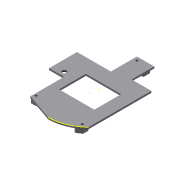
# Autodesk Inventor part: Raman2Go_Adapterplatte1_XY-TischChina
Saved by Autodesk Inventor 2019 (Build 230136000, 136)
## iProperties
Created: 2018-09-10
Part Number: Raman2Go_Adapterplatte1_XY-TischChina
Material: Generisch
Document SubType Name: Modeling
Designer: Henry John
Density: 1 g/cm^3
Appearance: Vorgabe
Author: Henry John
Autodesk Inventor part; units mm, degrees
ref_plane "YZ Plane" through (0, 0, 0) normal (1, 0, 0) x (0, 1, 0)
ref_plane "XZ Plane" through (0, 0, 0) normal (0, 1, 0) x (-1, 0, 0)
ref_plane "XY Plane" through (0, 0, 0) normal (0, 0, 1) x (1, 0, 0)
sketch "Skizze1" plane through (0, 0, 0) normal (0, 0, 1) x (1, 0, 0)
  circle A0 centre (-18.8292, -0.8203) radius 1.45 construction
  line L0 (-24.8792, -2.7703) -> (-24.8792, 8.6797) construction
  arc A1 (-11.8792, -25.2203) -> (6.3208, -26.6782) centre (-1.0025, -3.77) ccw construction
  circle A2 centre (-14.9792, -20.5703) radius 0.9 construction
  circle A3 centre (12.0208, -21.4394) radius 0.9 construction
  circle A4 centre (-3.6792, 25.2797) radius 0.9 construction
  line L1 (-5.6792, 27.2797) -> (3.4208, 27.2797) construction
  line L2 (25.1208, 7.4797) -> (25.1208, -1.5203) construction
  line L3 (25.1208, -27.8203) -> (-24.8792, -27.8203)
  line L4 (-24.8792, -27.8203) -> (-24.8792, 27.2797)
  line L5 (-24.8792, 27.2797) -> (25.1208, 27.2797)
  line L6 (25.1208, 27.2797) -> (25.1208, -27.8203)
  line L7 (4.6208, 0.2797) -> (4.6208, -6.9703) construction
  line L8 (-4.8792, 0.2797) -> (4.6208, 0.2797) construction
  line L9 (-4.8792, -6.9703) -> (-4.8792, 0.2797) construction
  line L10 (4.6208, -6.9703) -> (-4.8792, -6.9703) construction
  line L11 (-2.2292, 2.2797) -> (1.9708, 2.2797) construction
  line L12 (6.3708, 2.2797) -> (1.9708, 2.2797) construction
  line L13 (6.3708, -8.9703) -> (6.3708, 2.2797) construction
  line L14 (1.9708, -8.9703) -> (6.3708, -8.9703) construction
  line L15 (1.9708, -8.9703) -> (-2.2292, -8.9703) construction
  line L16 (-6.6292, -8.9703) -> (-2.2292, -8.9703) construction
  line L17 (-6.6292, 2.2797) -> (-6.6292, -8.9703) construction
  line L18 (-2.2292, 2.2797) -> (-6.6292, 2.2797) construction
  line L19 (-11.6292, -10.9703) -> (8.3708, -10.9703)
  line L20 (8.3708, -10.9703) -> (8.3708, 4.2797)
  line L21 (8.3708, 4.2797) -> (-11.6292, 4.2797)
  line L22 (-11.6292, 4.2797) -> (-11.6292, -10.9703)
  point P0 (0, 0)
  dimension "d48" = 2
  dimension "d49" = 2
  dimension "d50" = 2
  dimension "d51" = 5
  constraints: 16 end point, 4 parallel, 3 collinear, 2 horizontal, 2 perpendicular, 1 tangent
  measures "d48" distance between parallel lines of L20 L13
  measures "d49" distance between parallel lines of L18 L21
  measures "d50" distance between parallel lines of L15 L19
  measures "d51" distance between parallel lines of L17 L22
extrude "Extrusion1" add sketch "Skizze1" along normal blind 1
sketch "Skizze2" plane through (0, 0, 0) normal (0, 0, -1) x (-1, 0, 0)
  circle A0 centre (14.9792, -20.5703) radius 0.9 projected
  circle A1 centre (-12.0208, -21.4394) radius 0.9 construction
  circle A2 centre (3.6792, 25.2797) radius 0.9 construction
  circle A3 centre (14.9792, -20.5703) radius 0.9 projected
  circle A4 centre (9.7292, -19.9703) radius 0.75 projected
  line L0 (17.9792, -20.8203) -> (16.3292, -20.8203) construction
  line L1 (7.7292, -22.4703) -> (11.8792, -22.4703) construction
  line L2 (7.7292, -17.4703) -> (7.7292, -22.4703) construction
  line L3 (16.3292, -17.4703) -> (7.7292, -17.4703) construction
  line L4 (16.3292, -20.8203) -> (16.3292, -17.4703) construction
  line L5 (16.3292, -22.2703) -> (7.9292, -22.2703)
  line L6 (7.9292, -22.2703) -> (7.9292, -17.6703)
  line L7 (7.9292, -17.6703) -> (16.3292, -17.6703)
  line L8 (16.3292, -17.6703) -> (16.3292, -22.2703)
  line L9 (11.8792, -22.2703) -> (12.162, -22.2703) construction
  line L10 (16.3292, -17.6703) -> (12.3496, -17.6703)
  line L11 (12.3496, -17.6703) -> (12.3496, -22.2703)
  line L12 (12.3496, -22.2703) -> (16.3292, -22.2703)
  line L13 (16.3292, -22.2703) -> (16.3292, -17.6703)
  line L14 (16.3292, -22.2703) -> (13.494, -22.2703)
  line L15 (13.494, -22.2703) -> (13.494, -18.9379)
  line L16 (13.494, -18.9379) -> (16.3292, -18.9379)
  line L17 (16.3292, -18.9379) -> (16.3292, -22.2703)
  point P0 (0, 0)
  dimension "d3" = 0.2
  dimension "d4" = 0.2
  dimension "d9" = 0.2
  constraints: 26 end point, 5 parallel, 4 point on line, 3 horizontal, 2 perpendicular, 2 vertical, 1 vertical alignment
  measures "d3" distance between parallel lines of L3 L7
  measures "d4" distance between parallel lines of L2 L6
  measures "d9" distance between parallel lines of L5 L1
extrude "Extrusion2" add sketch "Skizze2" along normal blind 2.5 contours A0 | L5 L15 L16 L8
sketch "Skizze3" plane through (0, 0, -2.5) normal (0, 0, -1) x (-1, 0, 0)
  circle A0 centre (14.9792, -20.5703) radius 0.9 construction
  point P0 (0, 0)
hole "Bohrung1" at (-14.9792, -20.5703, -2.5) direction (0, 0, 1) diameter 1.221 depth 6.1 tip angle 118 thread size "M1.6x0.35" class "6H" standard "ISO Metric profile"
sketch "Skizze4" plane through (0, 0, 0) normal (0, 0, -1) x (-1, 0, 0)
  circle A0 centre (18.8292, -0.8203) radius 1.45 construction
  point P0 (0, 0)
hole "Bohrung2" at (-18.8292, -0.8203, 0) direction (0, 0, 1) diameter 2.459 end through all thread size "M3x0.5" class "6H" standard "ISO Metric profile"
sketch "Skizze5" plane through (0, 0, 0) normal (0, 0, -1) x (-1, 0, 0)
  line L0 (-9.3708, -21.4703) -> (-9.3708, -17.9703) construction
  line L1 (-14.1208, -16.9703) -> (-14.1208, -22.4703) construction
  line L2 (-15.3208, -16.9703) -> (-10.3708, -16.9703) construction
  line L3 (-9.3708, -17.9703) -> (-10.3708, -16.9703) construction
  line L4 (-9.3708, -21.4703) -> (-9.3708, -17.9703) construction
  line L5 (-10.5708, -16.9703) -> (-15.3208, -16.9703)
  line L6 (-15.3208, -16.9703) -> (-15.3208, -24.3394)
  line L7 (-15.3208, -24.3394) -> (-10.5708, -24.3394)
  line L8 (-10.5708, -24.3394) -> (-10.5708, -16.9703)
  line L9 (-15.3208, -16.9703) -> (-15.3208, -1.5203) construction
  circle A0 centre (-12.0208, -21.4394) radius 0.9 construction
  line L10 (-10.5708, -24.3394) -> (-13.7279, -24.3394)
  line L11 (-13.7279, -24.3394) -> (-13.7279, -16.9703)
  line L12 (-13.7279, -16.9703) -> (-10.5708, -16.9703)
  line L13 (-10.5708, -16.9703) -> (-10.5708, -24.3394)
  line L14 (-10.5708, -24.3394) -> (-13.7279, -24.3394)
  line L15 (-13.7279, -24.3394) -> (-13.7279, -19.7203)
  line L16 (-13.7279, -19.7203) -> (-10.5708, -19.7203)
  line L17 (-10.5708, -19.7203) -> (-10.5708, -24.3394)
  point P0 (0, 0)
extrude "Extrusion3" add sketch "Skizze5" along normal blind 2.3 contours L8 L7 L11 L16
sketch "Skizze6" plane through (0, 0, -2.3) normal (0, 0, -1) x (-1, 0, 0)
  circle A0 centre (-12.0208, -21.4394) radius 0.9 construction
  point P0 (0, 0)
hole "Bohrung3" at (12.0208, -21.4394, -2.3) direction (0, 0, 1) diameter 1.221 depth 7.1 tip angle 118 thread size "M1.6x0.35" class "6H" standard "ISO Metric profile"
sketch "Skizze7" plane through (0, 0, 0) normal (0, 0, -1) x (-1, 0, 0)
  circle A0 centre (3.6792, 25.2797) radius 0.9 construction
  line L0 (-3.4208, 24.7797) -> (-3.4208, 27.2797) construction
  line L1 (-1.9208, 24.7797) -> (-3.4208, 24.7797) construction
  line L2 (-1.9208, 23.2797) -> (-1.9208, 24.7797) construction
  line L3 (5.6792, 23.2797) -> (-1.9208, 23.2797) construction
  line L4 (5.6792, 27.2797) -> (5.6792, 23.2797) construction
  line L5 (-3.4208, 27.2797) -> (5.6792, 27.2797) construction
  line L6 (6.6792, 27.2797) -> (-1.7208, 27.2797)
  line L7 (-1.7208, 27.2797) -> (-1.7208, 23.4797)
  line L8 (-1.7208, 23.4797) -> (6.6792, 23.4797)
  line L9 (6.6792, 23.4797) -> (6.6792, 27.2797)
  point P0 (0, 0)
  dimension "d35" = 0.2
  dimension "d36" = 0.2
  dimension "d38" = 3
  constraints: 8 end point, 2 parallel, 1 collinear, 1 horizontal, 1 perpendicular
  measures "d35" distance between parallel lines of L3 L8
  measures "d36" distance between parallel lines of L7 L2
  measures "d38" distance from line of L9 A0.centre
extrude "Extrusion4" add sketch "Skizze7" along normal blind 3.5
sketch "Skizze8" plane through (0, 0, -3.5) normal (0, 0, -1) x (-1, 0, 0)
  circle A0 centre (3.6792, 25.2797) radius 0.9 construction
  point P0 (0, 0)
hole "Bohrung4" at (-3.6792, 25.2797, -3.5) direction (0, 0, 1) diameter 1.221 depth 7.1 tip angle 118 thread size "M1.6x0.35" class "6H" standard "ISO Metric profile"
sketch "Sketch9" plane through (0, 0, 1) normal (0, 0, 1) x (1, 0, 0)
  circle A0 centre (-18.8292, -0.8203) radius 1.45 construction
  line L0 (-22.6792, 10.4902) -> (-22.6792, -2.5703) construction
  line L1 (-22.6792, -2.5703) -> (-21.2792, -2.5703) construction
  line L2 (-21.2792, -2.5703) -> (-21.2792, 8.1297) construction
  arc A1 (-19.5792, 9.8297) -> (-21.2792, 8.1297) centre (-19.5792, 8.1297) ccw construction
  line L3 (-19.5792, 9.8297) -> (-13.5792, 9.8297) construction
  line L4 (-13.5792, 9.8297) -> (-13.5792, 11.4797) construction
  line L5 (-13.5792, 11.4797) -> (-22.1079, 11.4797) construction
  line L6 (-22.1079, 11.4797) -> (-22.6792, 10.4902) construction
  line L7 (-5.6792, 23.2797) -> (1.9208, 23.2797) construction
  line L8 (1.9208, 23.2797) -> (1.9208, 24.7797) construction
  line L9 (1.9208, 24.7797) -> (4.1208, 24.7797) construction
  line L10 (4.1208, 24.7797) -> (4.1208, 14.4797) construction
  line L11 (4.1208, 14.4797) -> (20.1208, 14.4797) construction
  line L12 (20.1208, 14.4797) -> (20.1208, 12.4797) construction
  line L13 (20.1208, 12.4797) -> (22.2341, 12.4797) construction
  line L14 (22.2341, 12.4797) -> (25.1208, 7.4797) construction
  line L15 (25.1208, 7.4797) -> (25.1208, -1.5203) construction
  line L16 (25.1208, -1.5203) -> (15.8208, -1.5203) construction
  line L17 (15.8208, -1.5203) -> (15.8208, -0.8203) construction
  line L18 (15.8208, -0.8203) -> (11.8208, -0.8203) construction
  line L19 (11.8208, -0.8203) -> (11.8208, -19.3203) construction
  line L20 (11.8208, -19.3203) -> (10.8208, -19.3203) construction
  line L21 (10.8208, -19.3203) -> (10.8208, 0.6797) construction
  line L22 (10.8208, 0.6797) -> (11.8208, 0.6797) construction
  line L23 (11.8208, 0.6797) -> (11.8208, 10.4297) construction
  line L24 (11.8208, 10.4297) -> (5.3208, 10.4297) construction
  line L25 (5.3208, 10.4297) -> (5.3208, 9.1297) construction
  line L26 (5.3208, 9.1297) -> (-19.5792, 9.1297) construction
  arc A2 (-19.5792, 9.1297) -> (-20.5792, 8.1297) centre (-19.5792, 8.1297) ccw construction
  line L27 (-20.5792, 8.1297) -> (-20.5792, 2.1297) construction
  arc A3 (-20.5792, 2.1297) -> (-20.0792, 1.6297) centre (-20.0792, 2.1297) ccw construction
  line L28 (-20.0792, 1.6297) -> (-18.8292, 1.6297) construction
  arc A4 (-16.3792, -0.8203) -> (-18.8292, 1.6297) centre (-18.8292, -0.8203) ccw construction
  line L29 (-16.3792, -0.8203) -> (-16.3792, -1.3703) construction
  arc A5 (-18.3792, -3.3703) -> (-16.3792, -1.3703) centre (-18.3792, -1.3703) ccw construction
  line L30 (-18.3792, -3.3703) -> (-23.4792, -3.3703) construction
  line L31 (-23.4792, -3.3703) -> (-23.4792, 11.1046) construction
  line L32 (-23.4792, 11.1046) -> (-22.6852, 12.4797) construction
  line L33 (-22.6852, 12.4797) -> (-13.6792, 12.4797) construction
  arc A6 (-13.6792, 12.4797) -> (-5.6792, 20.4797) centre (-13.6792, 20.4797) ccw construction
  line L34 (-5.6792, 20.4797) -> (-5.6792, 23.2797) construction
  line L35 (-7.8792, -20.1624) -> (-7.8792, -26.8162) construction
  arc A7 (-9.8792, -26.1222) -> (-7.8792, -26.8162) centre (-1.0025, -3.77) ccw construction
  line L36 (-9.8792, -26.1222) -> (-9.8792, -22.1222) construction
  line L37 (-9.8792, -22.1222) -> (-13.6811, -18.3203) construction
  line L38 (-13.6811, -18.3203) -> (-16.6811, -18.3203) construction
  line L39 (-16.6811, -18.3203) -> (-16.6811, -20.8203) construction
  line L40 (-24.8792, -20.8203) -> (-16.6811, -20.8203) construction
  line L41 (-24.8792, -3.3703) -> (-24.8792, -20.8203) construction
  line L42 (-18.3792, -3.3703) -> (-24.8792, -3.3703) construction
  arc A8 (-18.3792, -3.3703) -> (-16.3792, -1.3703) centre (-18.3792, -1.3703) ccw construction
  line L43 (-16.3792, -15.8703) -> (-16.3792, -1.3703) construction
  line L44 (-12.1713, -15.8703) -> (-16.3792, -15.8703) construction
  line L45 (-12.1713, -15.8703) -> (-7.8792, -20.1624) construction
  line L46 (9.3208, 7.5297) -> (11.8208, 7.5297) construction
  line L47 (11.8208, 0.6797) -> (11.8208, 7.5297) construction
  line L48 (10.8208, 0.6797) -> (11.8208, 0.6797) construction
  line L49 (10.8208, -19.3203) -> (10.8208, 0.6797) construction
  line L50 (11.8208, -19.3203) -> (10.8208, -19.3203) construction
  line L51 (11.8208, -0.8203) -> (11.8208, -19.3203) construction
  line L52 (15.8208, -0.8203) -> (11.8208, -0.8203) construction
  line L53 (15.8208, -1.5203) -> (15.8208, -0.8203) construction
  line L54 (15.3208, -1.5203) -> (15.8208, -1.5203) construction
  line L55 (15.3208, -16.9703) -> (15.3208, -1.5203) construction
  line L56 (14.1208, -16.9703) -> (15.3208, -16.9703) construction
  line L57 (14.1208, -20.2394) -> (14.1208, -16.9703) construction
  line L58 (14.1208, -20.2394) -> (13.6208, -20.2394) construction
  arc A9 (13.6208, -20.2394) -> (10.0208, -21.4394) centre (12.0208, -21.4394) ccw construction
  line L59 (10.0208, -21.4394) -> (10.0208, -25.1453) construction
  arc A10 (-1.5792, -27.8134) -> (10.0208, -25.1453) centre (-1.0025, -3.77) ccw construction
  line L60 (-1.5792, -27.8134) -> (-1.5792, -26.4134) construction
  line L61 (-1.5792, -26.4134) -> (0.4208, -26.4134) construction
  line L62 (0.4208, -26.4134) -> (0.9208, -25.9134) construction
  line L63 (0.9208, -25.9134) -> (2.9208, -25.9134) construction
  line L64 (2.9208, -25.9134) -> (3.4208, -25.4134) construction
  line L65 (3.4208, -25.4134) -> (5.4208, -25.4134) construction
  line L66 (5.4208, -25.4134) -> (9.0208, -21.8134) construction
  line L67 (9.0208, -21.8134) -> (9.0208, -19.0634) construction
  arc A11 (9.0208, -19.0634) -> (6.6502, -18.7996) centre (7.8502, -18.7996) ccw construction
  line L68 (6.6502, -18.7996) -> (6.6502, -17.7996) construction
  line L69 (6.6502, -17.7996) -> (2.1208, -13.2703) construction
  line L70 (2.1208, -13.2703) -> (-13.8792, -13.2703) construction
  line L71 (-13.8792, 0.1297) -> (-13.8792, -13.2703) construction
  arc A12 (-13.8792, 0.1297) -> (-15.8792, 2.1297) centre (-15.8792, 0.1297) ccw construction
  line L72 (-16.9792, 2.1297) -> (-15.8792, 2.1297) construction
  arc A13 (-17.9792, 3.1297) -> (-16.9792, 2.1297) centre (-16.9792, 3.1297) ccw construction
  line L73 (-17.9792, 4.5047) -> (-17.9792, 3.1297) construction
  arc A14 (-15.9792, 6.5047) -> (-17.9792, 4.5047) centre (-15.9792, 4.5047) ccw construction
  line L74 (-15.9792, 6.5047) -> (7.845, 6.5047) construction
  arc A15 (7.845, 6.5047) -> (9.3208, 7.5297) centre (9.3208, 5.9547) ccw construction
  line L75 (-2.2292, 2.2797) -> (-6.6292, 2.2797) construction
  line L76 (-6.6292, 2.2797) -> (-6.6292, -8.9703) construction
  line L77 (-6.6292, -8.9703) -> (-2.2292, -8.9703) construction
  line L78 (-2.2292, -8.9703) -> (-2.2292, -9.9953) construction
  line L79 (-2.2292, -9.9953) -> (1.9708, -9.9953) construction
  line L80 (1.9708, -9.9953) -> (1.9708, -8.9703) construction
  line L81 (1.9708, -8.9703) -> (6.3708, -8.9703) construction
  line L82 (6.3708, -8.9703) -> (6.3708, 2.2797) construction
  line L83 (6.3708, 2.2797) -> (1.9708, 2.2797) construction
  line L84 (1.9708, 2.2797) -> (1.9708, 3.3047) construction
  line L85 (1.9708, 3.3047) -> (-2.2292, 3.3047) construction
  line L86 (-2.2292, 3.3047) -> (-2.2292, 2.2797) construction
  circle A16 centre (-12.8292, 4.1297) radius 1.575 construction
  circle A17 centre (7.8502, -14.7996) radius 1.575 construction
  circle A18 centre (-15.8292, 4.1297) radius 0.75 construction
  line L87 (16.6208, -9.5203) -> (16.6208, -1.5203) construction
  line L88 (24.6208, -9.5203) -> (24.6208, -1.5203) construction
  circle A19 centre (-3.6792, 25.2797) radius 0.6105 projected
  circle A20 centre (12.0208, -21.4394) radius 0.6105 projected
  circle A21 centre (-18.8292, -0.8203) radius 1.2295 projected
  circle A22 centre (-14.9792, -20.5703) radius 0.6105 projected
  line L89 (-11.6292, -10.9703) -> (-11.6292, 4.2797) projected
  line L90 (-11.6292, 4.2797) -> (8.3708, 4.2797) projected
  line L91 (8.3708, 4.2797) -> (8.3708, -10.9703) projected
  line L92 (8.3708, -10.9703) -> (-11.6292, -10.9703) projected
  line L93 (-24.8792, -27.8203) -> (25.1208, -27.8203) projected
  line L94 (25.1208, -27.8203) -> (25.1208, 27.2797) projected
  line L95 (25.1208, 27.2797) -> (-24.8792, 27.2797) projected
  line L96 (-24.8792, 27.2797) -> (-24.8792, -27.8203) projected
  line L97 (25.1208, 27.2797) -> (25.1208, -27.8203) projected
  line L98 (25.1208, 27.2797) -> (4.1208, 27.2797)
  line L99 (4.1208, 27.2797) -> (4.1208, 14.4797)
  line L100 (4.1208, 14.4797) -> (25.1208, 14.4797)
  line L101 (25.1208, 14.4797) -> (25.1208, 27.2797)
  line L102 (-24.8792, 27.2797) -> (-6.6792, 27.2797) projected
  line L103 (-24.8792, 27.2797) -> (-5.6792, 27.2797)
  line L104 (-5.6792, 27.2797) -> (-5.6792, 12.4797)
  line L105 (-5.6792, 12.4797) -> (-24.8792, 12.4797)
  line L106 (-24.8792, 12.4797) -> (-24.8792, 27.2797)
  line L107 (25.1208, -27.8203) -> (15.3208, -27.8203)
  line L108 (15.3208, -27.8203) -> (15.3208, 14.4797)
  line L109 (15.3208, 14.4797) -> (25.1208, 14.4797)
  line L110 (25.1208, 14.4797) -> (25.1208, -27.8203)
  line L111 (-24.8792, -27.8203) -> (-16.3792, -27.8203)
  line L112 (-16.3792, -27.8203) -> (-16.3792, -3.3703)
  line L113 (-16.3792, -3.3703) -> (-24.8792, -3.3703)
  line L114 (-24.8792, -3.3703) -> (-24.8792, -27.8203)
  line L115 (-16.3292, -22.2703) -> (-7.9292, -22.2703) projected
  line L116 (15.3208, -16.9703) -> (15.3208, -24.3394) projected
  arc A23 (-16.3292, -22.2703) -> (15.3208, -21.1808) centre (-1.1083, -4.1747) ccw
  line L117 (-16.3292, -22.2703) -> (-16.3792, -22.2703)
  line L118 (25.1208, -27.8203) -> (-24.8792, -27.8203) projected
  line L119 (-7.9292, -22.2703) -> (-16.3292, -22.2703) projected
  line L120 (-16.3292, -22.2703) -> (-1.0025, -27.8203)
  point P0 (0, 0)
  point P1 (-21.6292, -3.3703)
  constraints: 40 end point, 8 parallel, 6 point on line, 5 coincident, 5 perpendicular, 4 horizontal, 4 point on circle, 2 vertical, 1 centre point, 1 midpoint, 4 other
extrude "Extrusion5" cut sketch "Sketch9" against normal blind 10 contours L96 L113 L112 L93 | A23 L108 L93 | L96 L95 L104 L105 | L108 L100 L94 L93 | L100 L99 L95 L94
sketch "Sketch11" plane through (0, 0, 1) normal (0, 0, 1) x (1, 0, 0)
  arc A0 (-1.0025, -27.8203) -> (15.3208, -21.1808) centre (-1.1083, -4.1747) ccw projected
  point P0 (0, 0)
sketch "Sketch12" plane through (0, 0, 1) normal (0, 0, 1) x (1, 0, 0)
  line L0 (-11.6292, -10.9703) -> (-11.6292, 4.2797) projected
  line L1 (-11.6292, 4.2797) -> (8.3708, 4.2797) projected
  line L2 (8.3708, 4.2797) -> (8.3708, -10.9703) projected
  line L3 (8.3708, -10.9703) -> (-11.6292, -10.9703) projected
  circle A0 centre (-14.9792, -20.5703) radius 0.6105 projected
  circle A1 centre (-18.8292, -0.8203) radius 1.2295 projected
  circle A2 centre (12.0208, -21.4394) radius 0.6105 projected
  circle A3 centre (-3.6792, 25.2797) radius 0.6105 projected
  arc A4 (-1.0025, -27.8203) -> (15.3208, -21.1808) centre (-1.1083, -4.1747) ccw projected
  line L4 (15.3208, -21.1808) -> (15.3208, 14.4797) projected
  line L5 (15.3208, 14.4797) -> (4.1208, 14.4797) projected
  line L6 (4.1208, 14.4797) -> (4.1208, 27.2797) projected
  line L7 (4.1208, 27.2797) -> (-5.6792, 27.2797) projected
  line L8 (-5.6792, 27.2797) -> (-5.6792, 12.4797) projected
  line L9 (-5.6792, 12.4797) -> (-24.8792, 12.4797) projected
  line L10 (-24.8792, 12.4797) -> (-24.8792, -3.3703) projected
  line L11 (-24.8792, -3.3703) -> (-16.3792, -3.3703) projected
  line L12 (-16.3792, -3.3703) -> (-16.3792, -27.8203) projected
  line L13 (-16.3792, -27.8203) -> (-1.0025, -27.8203) projected
  line L14 (-16.3292, -22.4703) -> (-17.9792, -20.8203) projected
  line L15 (-16.3792, -27.8203) -> (-1.0025, -27.8203) projected
  arc A5 (-1.0025, -27.8203) -> (15.3208, -21.1808) centre (-1.1083, -4.1747) ccw projected
  line L16 (-16.3292, -22.4703) -> (-1.0025, -27.8203)
  line L17 (-17.5522, -22.0433) -> (2.1832, -28.9323)
  line L18 (2.1832, -28.9323) -> (-1.056, -38.212)
  line L19 (-1.056, -38.212) -> (-20.7914, -31.323)
  line L20 (-20.7914, -31.323) -> (-17.5522, -22.0433)
  point P0 (0, 0)
  constraints: 10 end point, 2 parallel, 1 perpendicular, 1 point on line
extrude "Extrusion6" cut sketch "Sketch12" against normal blind 10 contours L17 L18 L19 L20 L12 L13 | L13 L12 L17 L16
